Autodesk Fusion 360 part; units mm, degrees
(part 9 of 13)
  line L7144 (95.2429, -95.2347) -> (95.2261, -95.2606)
  line L7145 (95.2114, -95.2876) -> (94.7288, -95.7702)
  line L7146 (112.501, -89.0386) -> (112.377, -88.9433)
  line L7147 (112.377, -88.9433) -> (112.282, -88.819)
  line L7148 (94.6404, -95.8068) -> (94.627, -95.8068)
  line L7149 (91.2502, -96.0114) -> (91.1387, -95.9546)
  line L7150 (94.627, -95.8068) -> (94.627, -96.0518)
  line L7151 (94.7, -95.7917) -> (94.6699, -95.7981)
  line L7152 (95.248, -95.1992) -> (95.2448, -95.2212)
  line L7153 (95.2438, -95.2283) -> (95.2429, -95.2347)
  line L7154 (94.627, -96.0518) -> (92.227, -96.0518)
  line L7155 (112.957, -89.0986) -> (112.801, -89.119)
  line L7156 (91.3739, -96.031) -> (91.2502, -96.0114)
  line L7157 (95.0012, -90.6052) -> (95.0009, -90.6006)
  line L7158 (97.3892, -88.1887) -> (97.3923, -88.1852)
  line L7159 (91.4975, -96.0114) -> (91.3739, -96.031)
  line L7160 (91.6975, -95.3959) -> (91.7543, -95.5074)
  line L7161 (111.572, -88.6389) -> (111.546, -88.6222)
  line L7162 (92.227, -95.5271) -> (92.227, -95.3118)
  line L7163 (97.395, -88.1844) -> (97.4002, -88.1805)
  line L7164 (90.9797, -95.5939) -> (90.9934, -95.5074)
  line L7165 (92.227, -96.0518) -> (92.227, -95.7771)
  line L7166 (90.9934, -95.5074) -> (91.0502, -95.3959)
  line L7167 (111.546, -88.6222) -> (111.519, -88.6074)
  line L7168 (97.3923, -88.1852) -> (97.395, -88.1844)
  line L7169 (94.7079, -95.787) -> (94.7052, -95.7878)
  line L7170 (95.248, -90.679) -> (95.248, -95.1992)
  line L7171 (111.519, -88.6074) -> (111.327, -88.4154)
  line L7172 (97.5116, -88.4154) -> (95.248, -90.679)
  line L7173 (111.327, -88.4154) -> (97.5116, -88.4154)
  line L7174 (90.9745, -95.716) -> (90.9597, -95.6472)
  line L7175 (91.0502, -95.8661) -> (90.9934, -95.7546)
  line L7176 (145.432, -71.1749) -> (145.598, -71.1574)
  line L7177 (95.2451, -95.2258) -> (95.2438, -95.2283)
  line L7178 (111.578, -88.6398) -> (111.572, -88.6389)
  line L7179 (91.6975, -95.8661) -> (91.609, -95.9546)
  line L7180 (94.627, -95.5184) -> (94.998, -95.1474)
  line L7181 (91.7488, -95.7653) -> (91.6975, -95.8661)
  line L7182 (91.7555, -95.5154) -> (92.227, -95.5271)
  line L7183 (96.127, -95.3118) -> (98.527, -95.3118)
  line L7184 (111.659, -88.394) -> (112.218, -88.394)
  line L7185 (102.348, -90.1491) -> (102.359, -90.2585)
  line L7186 (98.8989, -95.787) -> (98.8962, -95.7878)
  line L7187 (99.6056, -95.0844) -> (98.9198, -95.7702)
  line L7188 (92.227, -95.3118) -> (94.627, -95.3118)
  line L7189 (112.377, -88.0947) -> (112.501, -87.9994)
  line L7190 (98.527, -95.5568) -> (98.7796, -95.5568)
  line L7191 (112.646, -87.9394) -> (112.801, -87.919)
  line L7192 (102.341, -90.3274) -> (102.326, -90.3572)
  line L7193 (95.0009, -90.6006) -> (95.0022, -90.5981)
  line L7194 (102.308, -89.4086) -> (102.419, -89.4654)
  line L7195 (91.609, -95.3074) -> (91.6975, -95.3959)
  line L7196 (102.584, -89.789) -> (102.565, -89.9126)
  line L7197 (111.401, -88.1686) -> (111.406, -88.1683)
  line L7198 (97.4303, -88.1741) -> (97.4598, -88.1654)
  line L7199 (98.527, -95.8068) -> (98.527, -96.0518)
  line L7200 (91.2502, -95.2506) -> (91.3739, -95.231)
  line L7201 (98.8314, -95.8068) -> (98.527, -95.8068)
  line L7202 (98.527, -96.0518) -> (96.127, -96.0518)
  line L7203 (100.85, -93.7382) -> (99.6422, -94.9462)
  line L7204 (98.8609, -95.7981) -> (98.8314, -95.8068)
  line L7205 (111.467, -88.202) -> (111.659, -88.394)
  line L7206 (95.0198, -90.5658) -> (95.0346, -90.5388)
  line L7207 (102.419, -90.1126) -> (102.348, -90.1491)
  line L7208 (97.4002, -88.1805) -> (97.4303, -88.1741)
  line L7209 (91.7543, -95.5074) -> (91.7555, -95.5154)
  line L7210 (111.408, -88.1696) -> (111.415, -88.1705)
  line L7211 (111.415, -88.1705) -> (111.44, -88.1872)
  line L7212 (97.4598, -88.1654) -> (111.379, -88.1654)
  line L7213 (94.998, -90.6272) -> (95.0012, -90.6052)
  line L7214 (112.222, -88.3637) -> (112.282, -88.219)
  line L7215 (112.282, -88.219) -> (112.377, -88.0947)
  line L7216 (102.508, -89.5539) -> (102.565, -89.6654)
  line L7217 (112.218, -88.394) -> (112.222, -88.3637)
  line L7218 (102.565, -89.9126) -> (102.508, -90.0241)
  line L7219 (102.359, -90.2585) -> (102.358, -90.2944)
  line L7220 (111.406, -88.1683) -> (111.408, -88.1696)
  line L7221 (100.865, -93.7112) -> (100.85, -93.7382)
  line L7222 (94.627, -95.3118) -> (94.627, -95.5184)
  line L7223 (98.527, -95.3118) -> (98.527, -95.5568)
  line L7224 (100.882, -93.6853) -> (100.865, -93.7112)
  line L7225 (95.0346, -90.5388) -> (97.3714, -88.202)
  line L7226 (90.9934, -95.7546) -> (90.9908, -95.7378)
  line L7227 (112.501, -87.9994) -> (112.646, -87.9394)
  line L7228 (100.884, -93.6718) -> (100.884, -93.6764)
  line L7229 (99.639, -95.018) -> (99.6393, -95.0226)
  line L7230 (91.4975, -95.2506) -> (91.609, -95.3074)
  line L7231 (102.508, -90.0241) -> (102.419, -90.1126)
  line L7232 (102.358, -90.2944) -> (102.357, -90.2962)
  line L7233 (102.357, -90.2962) -> (102.357, -90.2982)
  line L7234 (102.419, -89.4654) -> (102.508, -89.5539)
  line L7235 (102.357, -90.2982) -> (102.341, -90.3274)
  line L7236 (91.0502, -95.3959) -> (91.1387, -95.3074)
  line L7237 (112.801, -87.919) -> (112.957, -87.9394)
  line L7238 (99.6393, -95.0226) -> (99.638, -95.0251)
  line L7239 (102.565, -89.6654) -> (102.584, -89.789)
  line L7240 (95.0031, -90.5917) -> (95.0198, -90.5658)
  line L7241 (111.44, -88.1872) -> (111.467, -88.202)
  line L7242 (102.326, -90.3572) -> (102.324, -90.3582)
  line L7243 (111.379, -88.1654) -> (111.401, -88.1686)
  line L7244 (98.902, -95.7835) -> (98.8989, -95.787)
  line L7245 (98.891, -95.7917) -> (98.8609, -95.7981)
  line L7246 (102.324, -90.3582) -> (102.323, -90.36)
  line L7247 (99.096, -94.3086) -> (99.123, -94.3234)
  line L7248 (126.104, -71.9283) -> (126.081, -72.0939)
  line L7249 (100.884, -93.6764) -> (100.883, -93.6789)
  line L7250 (102.061, -89.4086) -> (102.184, -89.389)
  line L7251 (129.614, -81.2299) -> (129.644, -81.2338)
  line L7252 (96.127, -94.0418) -> (98.527, -94.0418)
  line L7253 (101.949, -90.1126) -> (101.861, -90.0241)
  line L7254 (102.184, -89.389) -> (102.308, -89.4086)
  line L7255 (99.6422, -94.9462) -> (99.6422, -94.996)
  line L7256 (96.127, -94.7818) -> (96.127, -94.0418)
  line L7257 (102.099, -90.1755) -> (102.061, -90.1694)
  line L7258 (129.294, -75.6781) -> (129.301, -75.7082)
  line L7259 (99.0346, -94.2868) -> (99.0566, -94.29)
  line L7260 (101.949, -89.4654) -> (102.061, -89.4086)
  line L7261 (96.127, -96.0518) -> (96.127, -95.3118)
  line L7262 (99.6422, -94.996) -> (99.639, -95.018)
  line L7263 (98.527, -94.7818) -> (96.127, -94.7818)
  line L7264 (100.637, -91.7448) -> (100.64, -91.7228)
  line L7265 (100.64, -91.7228) -> (100.64, -91.7182)
  line L7266 (125.942, -71.4415) -> (126.03, -71.5833)
  line L7267 (125.683, -71.2333) -> (125.824, -71.3229)
  line L7268 (129.286, -75.6672) -> (129.29, -75.6702)
  line L7269 (98.8962, -95.7878) -> (98.891, -95.7917)
  line L7270 (99.0637, -94.291) -> (99.0701, -94.2919)
  line L7271 (99.638, -95.0251) -> (99.6371, -95.0315)
  line L7272 (129.578, -76.0608) -> (129.591, -76.0786)
  line L7273 (100.887, -91.7966) -> (100.887, -93.6498)
  line L7274 (100.64, -91.7182) -> (100.641, -91.7157)
  line L7275 (100.659, -91.6834) -> (100.673, -91.6564)
  line L7276 (101.861, -90.0241) -> (101.804, -89.9126)
  line L7277 (98.9828, -94.5368) -> (98.527, -94.5368)
  line L7278 (129.595, -76.0844) -> (129.599, -76.0896)
  line L7279 (100.887, -93.6498) -> (100.884, -93.6718)
  line L7280 (99.0701, -94.2919) -> (99.096, -94.3086)
  line L7281 (102.323, -90.36) -> (100.887, -91.7966)
  line L7282 (101.784, -89.789) -> (101.804, -89.6654)
  line L7283 (100.637, -93.598) -> (100.637, -91.7448)
  line L7284 (129.301, -75.7082) -> (129.309, -75.7377)
  line L7285 (129.606, -76.1197) -> (129.614, -76.1492)
  line L7286 (102.104, -90.2254) -> (102.099, -90.1755)
  line L7287 (98.9198, -95.7702) -> (98.902, -95.7835)
  line L7288 (125.962, -72.3388) -> (129.273, -75.6493)
  line L7289 (101.804, -89.9126) -> (101.784, -89.789)
  line L7290 (99.3912, -94.9452) -> (98.9828, -94.5368)
  line L7291 (98.527, -94.5368) -> (98.527, -94.7818)
  line L7292 (99.6371, -95.0315) -> (99.6204, -95.0574)
  line L7293 (129.614, -76.1492) -> (129.614, -81.2299)
  line L7294 (99.0612, -94.2897) -> (99.0637, -94.291)
  line L7295 (99.0566, -94.29) -> (99.0612, -94.2897)
  line L7296 (100.642, -91.7093) -> (100.659, -91.6834)
  line L7297 (102.061, -90.1694) -> (101.949, -90.1126)
  line L7298 (129.599, -76.0896) -> (129.606, -76.1197)
  line L7299 (100.673, -91.6564) -> (102.104, -90.2254)
  line L7300 (98.527, -94.0418) -> (98.527, -94.2868)
  line L7301 (129.591, -76.0786) -> (129.594, -76.0817)
  line L7302 (99.123, -94.3234) -> (99.5172, -94.7176)
  line L7303 (129.29, -75.6729) -> (129.294, -75.6781)
  line L7304 (98.527, -94.2868) -> (99.0346, -94.2868)
  line L7305 (98.7796, -95.5568) -> (99.3912, -94.9452)
  line L7306 (99.6204, -95.0574) -> (99.6056, -95.0844)
  line L7307 (100.883, -93.6789) -> (100.882, -93.6853)
  line L7308 (99.5172, -94.7176) -> (100.637, -93.598)
  line L7309 (100.641, -91.7157) -> (100.642, -91.7093)
  line L7310 (129.594, -76.0817) -> (129.595, -76.0844)
  line L7311 (128.91, -81.9687) -> (128.889, -81.8134)
  line L7312 (129.273, -75.6493) -> (129.286, -75.6672)
  line L7313 (125.525, -71.1772) -> (125.683, -71.2333)
  line L7314 (126.984, -94.7586) -> (126.873, -94.8154)
  line L7315 (130.089, -81.8134) -> (130.069, -81.9687)
  line L7316 (126.03, -71.5833) -> (126.085, -71.7412)
  line L7317 (130.069, -81.6581) -> (130.089, -81.8134)
  line L7318 (129.913, -81.3891) -> (130.009, -81.5134)
  line L7319 (129.364, -82.3969) -> (129.334, -82.393)
  line L7320 (126.369, -94.3114) -> (126.426, -94.1999)
  line L7321 (129.309, -75.7926) -> (129.578, -76.0608)
  line L7322 (129.614, -87.0204) -> (129.611, -87.0424)
  line L7323 (127.13, -94.3114) -> (127.149, -94.435)
  line L7324 (126.349, -94.435) -> (126.369, -94.3114)
  line L7325 (129.61, -87.0495) -> (129.609, -87.0559)
  line L7326 (127.073, -94.1999) -> (127.13, -94.3114)
  line L7327 (126.629, -89.7248) -> (126.646, -89.6989)
  line L7328 (126.626, -94.8154) -> (126.514, -94.7586)
  line L7329 (130.009, -82.1134) -> (129.913, -82.2377)
  line L7330 (126.624, -94.0553) -> (126.624, -89.7603)
  line L7331 (126.627, -89.7383) -> (126.627, -89.7337)
  line L7332 (126.646, -89.6989) -> (126.661, -89.6719)
  line L7333 (129.29, -75.6702) -> (129.29, -75.6729)
  line L7334 (129.644, -82.393) -> (129.614, -82.3969)
  line L7335 (127.13, -94.5586) -> (127.073, -94.6701)
  line L7336 (126.749, -94.835) -> (126.626, -94.8154)
  line L7337 (130.009, -81.5134) -> (130.069, -81.6581)
  line L7338 (101.861, -89.5539) -> (101.949, -89.4654)
  line L7339 (126.021, -72.2502) -> (125.962, -72.3388)
  line L7340 (126.081, -72.0939) -> (126.021, -72.2502)
  line L7341 (101.804, -89.6654) -> (101.861, -89.5539)
  line L7342 (126.984, -94.1114) -> (127.073, -94.1999)
  line L7343 (129.789, -82.333) -> (129.644, -82.393)
  line L7344 (126.874, -89.8121) -> (126.874, -94.0553)
  line L7345 (129.611, -87.0424) -> (129.611, -87.047)
  line L7346 (129.309, -75.7377) -> (129.309, -75.7926)
  line L7347 (129.592, -87.0818) -> (129.578, -87.1088)
  line L7348 (125.824, -71.3229) -> (125.942, -71.4415)
  line L7349 (129.614, -82.3969) -> (129.614, -87.0204)
  line L7350 (129.611, -87.047) -> (129.61, -87.0495)
  line L7351 (129.789, -81.2938) -> (129.913, -81.3891)
  line L7352 (129.913, -82.2377) -> (129.789, -82.333)
  line L7353 (126.627, -89.7337) -> (126.629, -89.7312)
  line L7354 (126.629, -89.7312) -> (126.629, -89.7248)
  line L7355 (126.085, -71.7412) -> (126.104, -71.9074)
  line L7356 (126.369, -94.5586) -> (126.349, -94.435)
  line L7357 (126.104, -71.9074) -> (126.104, -71.9283)
  line L7358 (130.069, -81.9687) -> (130.009, -82.1134)
  line L7359 (126.874, -94.0553) -> (126.984, -94.1114)
  line L7360 (127.149, -94.435) -> (127.13, -94.5586)
  line L7361 (126.514, -94.7586) -> (126.426, -94.6701)
  line L7362 (129.609, -87.0559) -> (129.592, -87.0818)
  line L7363 (128.889, -81.8134) -> (128.91, -81.6581)
  line L7364 (127.073, -94.6701) -> (126.984, -94.7586)
  line L7365 (129.189, -82.333) -> (129.065, -82.2377)
  line L7366 (129.065, -81.3891) -> (129.189, -81.2938)
  line L7367 (126.624, -89.7603) -> (126.627, -89.7383)
  line L7368 (129.578, -87.1088) -> (126.874, -89.8121)
  line L7369 (126.873, -94.8154) -> (126.749, -94.835)
  line L7370 (129.364, -86.9686) -> (129.364, -82.3969)
  line L7371 (129.189, -81.2938) -> (129.334, -81.2338)
  line L7372 (129.065, -82.2377) -> (128.97, -82.1134)
  line L7373 (129.644, -81.2338) -> (129.789, -81.2938)
  line L7374 (126.426, -94.1999) -> (126.514, -94.1114)
  line L7375 (130.867, -72.5048) -> (130.724, -72.5904)
  line L7376 (131.186, -85.0363) -> (131.207, -85.1916)
  line L7377 (124.673, -72.222) -> (124.62, -72.0633)
  line L7378 (125.193, -71.1749) -> (125.359, -71.1574)
  line L7379 (124.892, -71.3164) -> (125.035, -71.2288)
  line L7380 (129.334, -82.393) -> (129.189, -82.333)
  line L7381 (130.729, -87.1694) -> (130.729, -87.174)
  line L7382 (130.729, -87.174) -> (130.728, -87.1765)
  line L7383 (129.364, -81.2299) -> (129.364, -76.201)
  line L7384 (130.907, -84.672) -> (131.031, -84.7673)
  line L7385 (130.907, -85.7112) -> (130.762, -85.7712)
  line L7386 (130.762, -84.612) -> (130.907, -84.672)
  line L7387 (125.173, -72.6351) -> (125.016, -72.5768)
  line L7388 (125.664, -72.5904) -> (125.505, -72.6421)
  line L7389 (129.079, -75.9119) -> (129.078, -75.9092)
  line L7390 (124.773, -71.4334) -> (124.892, -71.3164)
  line L7391 (131.207, -85.1916) -> (131.186, -85.3469)
  line L7392 (131.164, -71.9074) -> (131.163, -71.9283)
  line L7393 (128.97, -82.1134) -> (128.91, -81.9687)
  line L7394 (130.884, -71.3229) -> (131.002, -71.4415)
  line L7395 (129.075, -75.904) -> (129.068, -75.8739)
  line L7396 (125.359, -71.1574) -> (125.525, -71.1772)
  line L7397 (124.62, -72.0633) -> (124.604, -71.8969)
  line L7398 (131.126, -85.4916) -> (131.031, -85.6159)
  line L7399 (129.059, -75.7895) -> (125.787, -72.5171)
  line L7400 (125.338, -72.6572) -> (125.173, -72.6351)
  line L7401 (129.334, -81.2338) -> (129.364, -81.2299)
  line L7402 (131.145, -71.7412) -> (131.164, -71.9074)
  line L7403 (130.539, -72.6444) -> (130.539, -84.6006)
  line L7404 (130.724, -72.5904) -> (130.565, -72.6421)
  line L7405 (129.083, -75.915) -> (129.079, -75.9119)
  line L7406 (130.743, -71.2333) -> (130.884, -71.3229)
  line L7407 (128.91, -81.6581) -> (128.97, -81.5134)
  line L7408 (130.585, -71.1772) -> (130.743, -71.2333)
  line L7409 (129.096, -75.9328) -> (129.083, -75.915)
  line L7410 (129.364, -76.201) -> (129.096, -75.9328)
  line L7411 (125.505, -72.6421) -> (125.338, -72.6572)
  line L7412 (124.76, -72.365) -> (124.673, -72.222)
  line L7413 (130.762, -85.7712) -> (130.732, -85.7751)
  line L7414 (131.081, -72.2502) -> (130.988, -72.3895)
  line L7415 (130.732, -85.7751) -> (130.732, -87.1474)
  line L7416 (131.031, -85.6159) -> (130.907, -85.7112)
  line L7417 (125.035, -71.2288) -> (125.193, -71.1749)
  line L7418 (126.661, -89.6719) -> (129.364, -86.9686)
  line L7419 (126.426, -94.6701) -> (126.369, -94.5586)
  line L7420 (124.682, -71.5739) -> (124.773, -71.4334)
  line L7421 (125.787, -72.5171) -> (125.664, -72.5904)
  line L7422 (129.078, -75.9092) -> (129.075, -75.904)
  line L7423 (129.059, -75.8444) -> (129.059, -75.7895)
  line L7424 (124.876, -72.4853) -> (124.76, -72.365)
  line L7425 (124.604, -71.8969) -> (124.625, -71.731)
  line L7426 (131.186, -85.3469) -> (131.126, -85.4916)
  line L7427 (129.068, -75.8739) -> (129.059, -75.8444)
  line L7428 (124.625, -71.731) -> (124.682, -71.5739)
  line L7429 (131.14, -72.0939) -> (131.081, -72.2502)
  line L7430 (126.514, -94.1114) -> (126.624, -94.0553)
  line L7431 (131.002, -71.4415) -> (131.09, -71.5833)
  line L7432 (128.97, -81.5134) -> (129.065, -81.3891)
  line L7433 (125.016, -72.5768) -> (124.876, -72.4853)
  line L7434 (130.565, -72.6421) -> (130.539, -72.6444)
  line L7435 (130.607, -84.5916) -> (130.762, -84.612)
  line L7436 (130.988, -72.3895) -> (130.867, -72.5048)
  line L7437 (131.126, -84.8916) -> (131.186, -85.0363)
  line L7438 (130.732, -87.1474) -> (130.729, -87.1694)
  line L7439 (130.728, -87.1765) -> (130.727, -87.1829)
  line L7440 (128.2, -93.7083) -> (128.22, -93.8319)
  line L7441 (128.144, -93.5968) -> (128.2, -93.7083)
  line L7442 (127.42, -93.8319) -> (127.44, -93.7083)
  line L7443 (128.055, -93.5083) -> (128.144, -93.5968)
  line L7444 (129.664, -71.8969) -> (129.685, -71.731)
  line L7445 (127.496, -94.0671) -> (127.44, -93.9555)
  line L7446 (130.027, -85.3469) -> (130.007, -85.1916)
  line L7447 (127.945, -89.9859) -> (127.945, -93.4522)
  line L7448 (130.087, -85.4916) -> (130.027, -85.3469)
  line L7449 (127.585, -94.1555) -> (127.496, -94.0671)
  line L7450 (130.183, -85.6159) -> (130.087, -85.4916)
  line L7451 (92.227, -93.0168) -> (92.227, -92.7718)
  line L7452 (127.585, -93.5083) -> (127.695, -93.4522)
  line L7453 (128.2, -93.9555) -> (128.144, -94.0671)
  line L7454 (128.055, -94.1555) -> (127.944, -94.2124)
  line L7455 (130.539, -84.6006) -> (130.607, -84.5916)
  line L7456 (127.944, -94.2124) -> (127.82, -94.2319)
  line L7457 (127.698, -89.9121) -> (127.698, -89.9075)
  line L7458 (130.289, -84.6858) -> (130.289, -72.6427)
  line L7459 (128.22, -93.8319) -> (128.2, -93.9555)
  line L7460 (131.09, -71.5833) -> (131.145, -71.7412)
  line L7461 (130.482, -87.0956) -> (130.482, -85.7751)
  line L7462 (130.727, -87.1829) -> (130.71, -87.2088)
  line L7463 (131.163, -71.9283) -> (131.14, -72.0939)
  line L7464 (127.698, -89.9075) -> (127.699, -89.905)
  line L7465 (127.717, -89.8728) -> (127.732, -89.8457)
  line L7466 (131.031, -84.7673) -> (131.126, -84.8916)
  line L7467 (127.945, -93.4522) -> (128.055, -93.5083)
  line L7468 (130.695, -87.2358) -> (127.945, -89.9859)
  line L7469 (127.44, -93.7083) -> (127.496, -93.5968)
  line L7470 (127.695, -93.4522) -> (127.695, -89.9341)
  line L7471 (128.144, -94.0671) -> (128.055, -94.1555)
  line L7472 (127.496, -93.5968) -> (127.585, -93.5083)
  line L7473 (130.71, -87.2088) -> (130.695, -87.2358)
  line L7474 (127.695, -89.9341) -> (127.698, -89.9121)
  line L7475 (127.696, -94.2124) -> (127.585, -94.1555)
  line L7476 (130.482, -85.7751) -> (130.452, -85.7712)
  line L7477 (127.7, -89.8986) -> (127.717, -89.8728)
  line L7478 (127.699, -89.905) -> (127.7, -89.8986)
  line L7479 (130.452, -85.7712) -> (130.307, -85.7112)
  line L7480 (127.44, -93.9555) -> (127.42, -93.8319)
  line L7481 (130.087, -84.8916) -> (130.183, -84.7673)
  line L7482 (98.527, -93.5118) -> (96.127, -93.5118)
  line L7483 (96.127, -93.5118) -> (96.127, -92.7718)
  line L7484 (130.307, -85.7112) -> (130.183, -85.6159)
  line L7485 (90.2188, -92.3788) -> (90.8568, -93.0168)
  line L7486 (129.685, -71.731) -> (129.742, -71.5739)
  line L7487 (127.82, -94.2319) -> (127.696, -94.2124)
  line L7488 (127.732, -89.8457) -> (130.482, -87.0956)
  line L7489 (90.8568, -93.0168) -> (92.227, -93.0168)
  line L7490 (89.9878, -92.4954) -> (89.9839, -92.4902)
  line L7491 (130.007, -85.1916) -> (130.027, -85.0363)
  line L7492 (96.127, -92.7718) -> (98.527, -92.7718)
  line L7493 (89.9886, -92.4981) -> (89.9878, -92.4954)
  line L7494 (129.936, -72.4853) -> (129.82, -72.365)
  line L7495 (90.7436, -93.245) -> (90.7166, -93.2302)
  line L7496 (89.9688, -91.1098) -> (89.972, -91.0878)
  line L7497 (93.1076, -87.9265) -> (93.1377, -87.9201)
  line L7498 (90.7695, -93.2617) -> (90.7436, -93.245)
  line L7499 (92.227, -93.2668) -> (90.805, -93.2668)
  line L7500 (90.783, -93.2636) -> (90.7784, -93.2639)
  line L7501 (90.7166, -93.2302) -> (90.0054, -92.519)
  line L7502 (129.742, -71.5739) -> (129.833, -71.4334)
  line L7503 (130.094, -71.2288) -> (130.253, -71.1749)
  line L7504 (98.527, -92.7718) -> (98.527, -93.5118)
  line L7505 (130.253, -71.1749) -> (130.419, -71.1574)
  line L7506 (93.1024, -87.9304) -> (93.1076, -87.9265)
  line L7507 (90.7784, -93.2639) -> (90.7759, -93.2626)
  line L7508 (89.9717, -91.0832) -> (89.973, -91.0807)
  line L7509 (94.627, -92.7718) -> (94.627, -93.5118)
  line L7510 (129.68, -72.0633) -> (129.664, -71.8969)
  line L7511 (129.82, -72.365) -> (129.733, -72.222)
  line L7512 (90.0054, -91.0214) -> (93.0788, -87.948)
  line L7513 (129.833, -71.4334) -> (129.952, -71.3164)
  line L7514 (130.076, -72.5768) -> (129.936, -72.4853)
  line L7515 (129.952, -71.3164) -> (130.094, -71.2288)
  line L7516 (130.289, -72.6427) -> (130.232, -72.6351)
  line L7517 (93.1377, -87.9201) -> (93.1672, -87.9114)
  line L7518 (95.249, -87.9114) -> (96.5308, -86.6297)
  line L7519 (93.1672, -87.9114) -> (95.249, -87.9114)
  line L7520 (94.627, -93.5118) -> (92.227, -93.5118)
  line L7521 (93.0997, -87.9312) -> (93.1024, -87.9304)
  line L7522 (90.805, -93.2668) -> (90.783, -93.2636)
  line L7523 (130.027, -85.0363) -> (130.087, -84.8916)
  line L7524 (130.419, -71.1574) -> (130.585, -71.1772)
  line L7525 (89.9688, -92.4306) -> (89.9688, -91.1098)
  line L7526 (92.227, -93.5118) -> (92.227, -93.2668)
  line L7527 (89.9739, -91.0743) -> (89.9906, -91.0484)
  line L7528 (92.227, -92.7718) -> (94.627, -92.7718)
  line L7529 (93.0788, -87.948) -> (93.0966, -87.9347)
  line L7530 (89.9775, -92.4601) -> (89.9688, -92.4306)
  line L7531 (130.232, -72.6351) -> (130.076, -72.5768)
  line L7532 (89.972, -91.0878) -> (89.9717, -91.0832)
  line L7533 (129.733, -72.222) -> (129.68, -72.0633)
  line L7534 (89.9921, -92.5012) -> (89.9886, -92.4981)
  line L7535 (89.973, -91.0807) -> (89.9739, -91.0743)
  line L7536 (90.7759, -93.2626) -> (90.7695, -93.2617)
  line L7537 (93.0966, -87.9347) -> (93.0997, -87.9312)
  line L7538 (130.183, -84.7673) -> (130.289, -84.6858)
  line L7539 (89.9906, -91.0484) -> (90.0054, -91.0214)
  line L7540 (123.432, -92.4354) -> (123.528, -92.3111)
  line L7541 (120.78, -92.105) -> (120.925, -92.165)
  line L7542 (124.552, -92.7354) -> (124.532, -92.8907)
  line L7543 (96.5308, -86.6297) -> (96.4952, -86.5598)
  line L7544 (96.6405, -86.1126) -> (96.752, -86.0558)
  line L7545 (97.1107, -86.7598) -> (96.9992, -86.8166)
  line L7546 (96.4952, -86.3126) -> (96.552, -86.2011)
  line L7547 (96.8756, -86.8362) -> (96.752, -86.8166)
  line L7548 (95.3656, -88.1424) -> (95.3604, -88.1463)
  line L7549 (95.3604, -88.1463) -> (95.3303, -88.1527)
  line L7550 (120.78, -93.2642) -> (120.625, -93.2846)
  line L7551 (97.2756, -86.4362) -> (97.256, -86.5598)
  line L7552 (124.252, -93.255) -> (124.107, -93.315)
  line L7553 (96.752, -86.0558) -> (96.8756, -86.0362)
  line L7554 (96.7158, -86.7982) -> (95.3892, -88.1248)
  line L7555 (97.1107, -86.1126) -> (97.1992, -86.2011)
  line L7556 (95.3683, -88.1416) -> (95.3656, -88.1424)
  line L7557 (124.472, -93.0354) -> (124.376, -93.1597)
  line L7558 (96.552, -86.2011) -> (96.6405, -86.1126)
  line L7559 (124.107, -93.315) -> (123.952, -93.3354)
  line L7560 (97.256, -86.5598) -> (97.1992, -86.6713)
  line L7561 (123.372, -92.8907) -> (123.352, -92.7354)
  line L7562 (124.376, -92.3111) -> (124.472, -92.4354)
  line L7563 (123.952, -92.1354) -> (124.107, -92.1558)
  line L7564 (96.752, -86.8166) -> (96.7158, -86.7982)
  line L7565 (123.952, -93.3354) -> (123.797, -93.315)
  line L7566 (97.256, -86.3126) -> (97.2756, -86.4362)
  line L7567 (90.2188, -91.1616) -> (90.2188, -92.3788)
  line L7568 (123.797, -92.1558) -> (123.952, -92.1354)
  line L7569 (123.652, -92.2158) -> (123.797, -92.1558)
  line L7570 (120.925, -92.165) -> (121.049, -92.2603)
  line L7571 (121.049, -92.2603) -> (121.144, -92.3846)
  line L7572 (90.0054, -92.519) -> (89.9921, -92.5012)
  line L7573 (95.3714, -88.1381) -> (95.3683, -88.1416)
  line L7574 (96.4756, -86.4362) -> (96.4952, -86.3126)
  line L7575 (95.3008, -88.1614) -> (93.219, -88.1614)
  line L7576 (124.252, -92.2158) -> (124.376, -92.3111)
  line L7577 (121.225, -92.6846) -> (121.204, -92.8399)
  line L7578 (95.3892, -88.1248) -> (95.3714, -88.1381)
  line L7579 (96.8756, -86.0362) -> (96.9992, -86.0558)
  line L7580 (89.9839, -92.4902) -> (89.9775, -92.4601)
  line L7581 (97.1992, -86.6713) -> (97.1107, -86.7598)
  line L7582 (95.3303, -88.1527) -> (95.3008, -88.1614)
  line L7583 (97.1992, -86.2011) -> (97.256, -86.3126)
  line L7584 (124.532, -92.8907) -> (124.472, -93.0354)
  line L7585 (96.4952, -86.5598) -> (96.4756, -86.4362)
  line L7586 (96.9992, -86.0558) -> (97.1107, -86.1126)
  line L7587 (93.219, -88.1614) -> (90.2188, -91.1616)
  line L7588 (120.925, -93.2042) -> (120.78, -93.2642)
  line L7589 (96.9992, -86.8166) -> (96.8756, -86.8362)
  line L7590 (121.144, -92.9846) -> (121.049, -93.1089)
  line L7591 (121.144, -92.3846) -> (121.204, -92.5293)
  line L7592 (121.204, -92.5293) -> (121.225, -92.6846)
  line L7593 (124.376, -93.1597) -> (124.252, -93.255)
  line L7594 (124.107, -92.1558) -> (124.252, -92.2158)
  line L7595 (121.049, -93.1089) -> (120.925, -93.2042)
  line L7596 (136.044, -87.344) -> (136.056, -87.3434)
  line L7597 (137.219, -85.9102) -> (137.286, -85.9336)
  line L7598 (124.472, -92.4354) -> (124.532, -92.5801)
  line L7599 (136.257, -87.3131) -> (136.439, -87.2514)
  line L7600 (121.204, -92.8399) -> (121.144, -92.9846)
  line L7601 (120.2, -92.2603) -> (120.325, -92.165)
  line L7602 (120.045, -92.8399) -> (120.025, -92.6846)
  line L7603 (120.045, -92.5293) -> (120.105, -92.3846)
  line L7604 (136.571, -86.3883) -> (136.552, -86.4343)
  line L7605 (137.15, -85.9267) -> (137.219, -85.9102)
  line L7606 (136.571, -86.0777) -> (136.592, -86.233)
  line L7607 (135.642, -87.289) -> (135.653, -87.2926)
  line L7608 (123.372, -92.5801) -> (123.432, -92.4354)
  line L7609 (137.102, -86.2949) -> (137.103, -86.2875)
  line L7610 (135.331, -87.3466) -> (135.351, -87.2784)
  line L7611 (136.246, -87.3158) -> (136.257, -87.3131)
  line L7612 (120.105, -92.9846) -> (120.045, -92.8399)
  line L7613 (136.941, -86.8059) -> (137.005, -86.6906)
  line L7614 (137.005, -86.6906) -> (137.01, -86.6801)
  line L7615 (120.469, -92.105) -> (120.625, -92.0846)
  line L7616 (123.797, -93.315) -> (123.652, -93.255)
  line L7617 (123.352, -92.7354) -> (123.372, -92.5801)
  line L7618 (120.625, -92.0846) -> (120.78, -92.105)
  line L7619 (120.105, -92.3846) -> (120.2, -92.2603)
  line L7620 (136.416, -85.8087) -> (136.511, -85.933)
  line L7621 (136.592, -86.233) -> (136.571, -86.3883)
  line L7622 (120.325, -92.165) -> (120.469, -92.105)
  line L7623 (136.292, -85.7134) -> (136.416, -85.8087)
  line L7624 (135.475, -87.2218) -> (135.507, -87.2308)
  line L7625 (137.103, -86.2875) -> (137.104, -86.2367)
  line L7626 (123.432, -93.0354) -> (123.372, -92.8907)
  line L7627 (137.104, -86.2293) -> (137.087, -86.0475)
  line L7628 (135.331, -92.6423) -> (135.331, -87.3466)
  line L7629 (137.447, -92.1893) -> (137.427, -92.2574)
  line L7630 (137.286, -85.9336) -> (137.302, -85.9469)
  line L7631 (136.147, -85.6534) -> (136.292, -85.7134)
  line L7632 (124.532, -92.5801) -> (124.552, -92.7354)
  line L7633 (123.652, -93.255) -> (123.528, -93.1597)
  line L7634 (120.2, -93.1089) -> (120.105, -92.9846)
  line L7635 (120.325, -93.2042) -> (120.2, -93.1089)
  line L7636 (135.343, -92.6946) -> (135.331, -92.6423)
  line L7637 (137.302, -85.9469) -> (137.41, -86.055)
  line L7638 (136.957, -92.7314) -> (136.895, -92.7654)
  line L7639 (137.104, -86.2367) -> (137.104, -86.2293)
  line L7640 (137.41, -92.2784) -> (136.957, -92.7314)
  line L7641 (123.528, -93.1597) -> (123.432, -93.0354)
  line L7642 (136.511, -85.933) -> (136.571, -86.0777)
  line L7643 (136.934, -86.8108) -> (136.941, -86.8059)
  line L7644 (137.072, -86.4982) -> (137.074, -86.487)
  line L7645 (137.074, -86.487) -> (137.102, -86.2949)
  line L7646 (120.625, -93.2846) -> (120.469, -93.2642)
  line L7647 (136.922, -86.804) -> (136.934, -86.8108)
  line L7648 (136.056, -87.3434) -> (136.246, -87.3158)
  line L7649 (123.528, -92.3111) -> (123.652, -92.2158)
  line L7650 (137.01, -86.6801) -> (137.072, -86.4982)
  line L7651 (136.552, -86.4343) -> (136.922, -86.804)
  line L7652 (137.427, -92.2574) -> (137.41, -92.2784)
  line L7653 (120.025, -92.6846) -> (120.045, -92.5293)
  line L7654 (135.351, -87.2784) -> (135.405, -87.2319)
  line L7655 (135.852, -87.3365) -> (136.044, -87.344)
  line L7656 (135.507, -87.2308) -> (135.642, -87.289)
  line L7657 (135.405, -87.2319) -> (135.475, -87.2218)
  line L7658 (120.469, -93.2642) -> (120.325, -93.2042)
  line L7659 (137.447, -86.1441) -> (137.447, -92.1893)
  line L7660 (112.468, -84.0786) -> (112.624, -84.0582)
  line L7661 (112.624, -84.0582) -> (112.779, -84.0786)
  line L7662 (112.104, -84.9582) -> (112.044, -84.8135)
  line L7663 (91.502, -91.9968) -> (91.4588, -92.0815)
  line L7664 (111.685, -83.5709) -> (111.688, -83.5722)
  line L7665 (135.412, -86.3883) -> (135.392, -86.233)
  line L7666 (135.392, -86.233) -> (135.412, -86.0777)
  line L7667 (135.567, -86.6573) -> (135.472, -86.533)
  line L7668 (135.692, -85.7134) -> (135.836, -85.6534)
  line L7669 (136.147, -86.8126) -> (135.992, -86.833)
  line L7670 (111.68, -83.5712) -> (111.685, -83.5709)
  line L7671 (91.4588, -92.0815) -> (91.3703, -92.17)
  line L7672 (112.924, -85.1778) -> (112.779, -85.2378)
  line L7673 (135.457, -92.7683) -> (135.389, -92.7483)
  line L7674 (111.747, -83.6046) -> (112.299, -84.1572)
  line L7675 (112.324, -85.1778) -> (112.199, -85.0825)
  line L7676 (112.104, -84.3582) -> (112.123, -84.334)
  line L7677 (136.193, -86.7935) -> (136.147, -86.8126)
  line L7678 (94.627, -92.2418) -> (92.227, -92.2418)
  line L7679 (91.2588, -92.2268) -> (91.1352, -92.2464)
  line L7680 (135.567, -85.8087) -> (135.692, -85.7134)
  line L7681 (135.389, -92.7483) -> (135.343, -92.6946)
  line L7682 (112.324, -84.1386) -> (112.468, -84.0786)
  line L7683 (136.449, -87.2467) -> (136.56, -87.1849)
  line L7684 (111.72, -83.5898) -> (111.747, -83.6046)
  line L7685 (135.841, -87.335) -> (135.852, -87.3365)
  line L7686 (137.101, -85.9779) -> (137.15, -85.9267)
  line L7687 (137.41, -86.055) -> (137.444, -86.1173)
  line L7688 (137.444, -86.1173) -> (137.447, -86.1441)
  line L7689 (137.087, -86.0475) -> (137.101, -85.9779)
  line L7690 (135.653, -87.2926) -> (135.841, -87.335)
  line L7691 (135.836, -86.8126) -> (135.692, -86.7526)
  line L7692 (136.56, -87.1849) -> (136.569, -87.1748)
  line L7693 (112.924, -84.1386) -> (113.048, -84.2339)
  line L7694 (136.569, -87.1748) -> (136.567, -87.1671)
  line L7695 (136.868, -92.7683) -> (135.457, -92.7683)
  line L7696 (135.412, -86.0777) -> (135.472, -85.933)
  line L7697 (112.779, -84.0786) -> (112.924, -84.1386)
  line L7698 (111.688, -83.5722) -> (111.694, -83.5731)
  line L7699 (135.472, -85.933) -> (135.567, -85.8087)
  line L7700 (135.836, -85.6534) -> (135.992, -85.633)
  line L7701 (111.694, -83.5731) -> (111.72, -83.5898)
  line L7702 (135.992, -85.633) -> (136.147, -85.6534)
  line L7703 (136.567, -87.1671) -> (136.193, -86.7935)
  line L7704 (135.692, -86.7526) -> (135.567, -86.6573)
  line L7705 (92.227, -91.9968) -> (91.502, -91.9968)
  line L7706 (135.472, -86.533) -> (135.412, -86.3883)
  line L7707 (136.439, -87.2514) -> (136.449, -87.2467)
  line L7708 (136.895, -92.7654) -> (136.868, -92.7683)
  line L7709 (135.992, -86.833) -> (135.836, -86.8126)
  line L7710 (91.3703, -92.17) -> (91.2588, -92.2268)
  line L7711 (112.299, -84.1572) -> (112.324, -84.1386)
  line L7712 (97.9182, -122.179) -> (97.8258, -122.026)
  line L7713 (105.074, -138.481) -> (105.006, -138.58)
  line L7714 (103.998, -138.006) -> (103.993, -138.004)
  line L7715 (107.336, -138.577) -> (107.295, -138.513)
  line L7716 (97.8354, -121.335) -> (97.932, -121.185)
  line L7717 (147.672, -102.363) -> (147.784, -102.419)
  line L7718 (99.179, -121.194) -> (99.2735, -121.345)
  line L7719 (99.3269, -121.89) -> (99.2635, -122.056)
  line L7720 (98.9027, -120.972) -> (99.0533, -121.067)
  line L7721 (98.2114, -120.967) -> (98.3802, -120.909)
  line L7722 (99.352, -121.691) -> (99.3517, -121.713)
  line L7723 (101.752, -123.609) -> (101.758, -123.614)
  line L7724 (108.078, -129.982) -> (108.078, -138.036)
  line L7725 (97.7695, -121.857) -> (97.7521, -121.679)
  line L7726 (99.0357, -122.328) -> (98.8825, -122.419)
  line L7727 (97.8258, -122.026) -> (97.7695, -121.857)
  line L7728 (99.3321, -121.513) -> (99.352, -121.691)
  line L7729 (98.3802, -120.909) -> (98.5576, -120.891)
  line L7730 (108.042, -129.892) -> (108.076, -129.955)
  line L7731 (99.1648, -122.205) -> (99.0357, -122.328)
  line L7732 (107.955, -138.178) -> (107.877, -138.236)
  line L7733 (99.2735, -121.345) -> (99.3321, -121.513)
  line L7734 (99.3517, -121.713) -> (99.3269, -121.89)
  line L7735 (98.1913, -122.405) -> (98.0421, -122.307)
  line L7736 (104.621, -138.364) -> (104.596, -138.337)
  line L7737 (104.41, -138.191) -> (104.216, -138.084)
  line L7738 (98.8825, -122.419) -> (98.7129, -122.474)
  line L7739 (104.418, -138.197) -> (104.414, -138.193)
  line L7740 (103.988, -138.003) -> (103.832, -137.975)
  line L7741 (97.932, -121.185) -> (98.0595, -121.06)
  line L7742 (104.414, -138.193) -> (104.41, -138.191)
  line L7743 (147.929, -102.619) -> (147.949, -102.743)
  line L7744 (105.415, -138.178) -> (105.313, -138.254)
  line L7745 (104.418, -138.197) -> (104.418, -138.197)
  line L7746 (98.5352, -122.49) -> (98.3585, -122.467)
  line L7747 (103.998, -138.006) -> (103.998, -138.006)
  line L7748 (97.7521, -121.679) -> (97.7744, -121.502)
  line L7749 (97.7744, -121.502) -> (97.8354, -121.335)
  line L7750 (98.0595, -121.06) -> (98.2114, -120.967)
  line L7751 (99.0533, -121.067) -> (99.179, -121.194)
  line L7752 (98.3585, -122.467) -> (98.1913, -122.405)
  line L7753 (98.7129, -122.474) -> (98.5352, -122.49)
  line L7754 (147.872, -102.508) -> (147.929, -102.619)
  line L7755 (99.2635, -122.056) -> (99.1648, -122.205)
  line L7756 (98.5576, -120.891) -> (98.7347, -120.912)
  line L7757 (98.0421, -122.307) -> (97.9182, -122.179)
  line L7758 (147.784, -102.419) -> (147.872, -102.508)
  line L7759 (104.755, -138.513) -> (104.752, -138.508)
  line L7760 (102.752, -139.183) -> (102.81, -139.005)
  line L7761 (102.752, -139.558) -> (102.732, -139.371)
  line L7762 (104.592, -138.334) -> (104.592, -138.334)
  line L7763 (104.796, -138.577) -> (104.755, -138.513)
  line L7764 (102.81, -139.737) -> (102.752, -139.558)
  line L7765 (104.082, -140.15) -> (103.91, -140.227)
  line L7766 (103.993, -138.004) -> (103.988, -138.003)
  line L7767 (104.36, -138.842) -> (104.454, -139.005)
  line L7768 (104.817, -138.602) -> (104.796, -138.577)
  line L7769 (103.03, -140.039) -> (102.904, -139.9)
  line L7770 (102.81, -139.005) -> (102.904, -138.842)
  line L7771 (104.951, -138.625) -> (104.881, -138.633)
  line L7772 (103.832, -138.498) -> (103.91, -138.515)
  line L7773 (104.206, -138.08) -> (104.206, -138.08)
  line L7774 (102.732, -139.371) -> (102.752, -139.183)
  line L7775 (105.313, -138.254) -> (105.234, -138.314)
  line L7776 (104.234, -140.039) -> (104.082, -140.15)
  line L7777 (102.904, -138.842) -> (103.03, -138.702)
  line L7778 (104.592, -138.334) -> (104.418, -138.197)
  line L7779 (103.988, -138.003) -> (103.988, -138.003)
  line L7780 (103.91, -140.227) -> (103.726, -140.266)
  line L7781 (105.006, -138.58) -> (104.951, -138.625)
  line L7782 (103.538, -140.266) -> (103.354, -140.227)
  line L7783 (103.182, -140.15) -> (103.03, -140.039)
  line L7784 (104.512, -139.183) -> (104.532, -139.371)
  line L7785 (104.732, -138.487) -> (104.621, -138.364)
  line L7786 (104.211, -138.081) -> (104.206, -138.08)
  line L7787 (104.512, -139.558) -> (104.454, -139.737)
  line L7788 (104.216, -138.084) -> (104.211, -138.081)
  line L7789 (103.354, -140.227) -> (103.182, -140.15)
  line L7790 (104.41, -138.191) -> (104.41, -138.191)
  line L7791 (104.596, -138.337) -> (104.592, -138.334)
  line L7792 (102.904, -139.9) -> (102.81, -139.737)
  line L7793 (103.91, -138.515) -> (104.082, -138.591)
  line L7794 (104.881, -138.633) -> (104.817, -138.602)
  line L7795 (103.726, -140.266) -> (103.538, -140.266)
  line L7796 (103.182, -138.591) -> (103.354, -138.515)
  line L7797 (104.532, -139.371) -> (104.512, -139.558)
  line L7798 (103.03, -138.702) -> (103.182, -138.591)
  line L7799 (104.206, -138.08) -> (103.998, -138.006)
  line L7800 (105.234, -138.314) -> (105.074, -138.481)
  line L7801 (104.36, -139.9) -> (104.234, -140.039)
  line L7802 (104.752, -138.508) -> (104.732, -138.487)
  line L7803 (105.415, -138.178) -> (105.415, -138.178)
  line L7804 (104.454, -139.737) -> (104.36, -139.9)
  line L7805 (104.216, -138.084) -> (104.216, -138.084)
  line L7806 (103.354, -138.515) -> (103.432, -138.498)
  line L7807 (103.432, -138.498) -> (103.432, -137.976)
  line L7808 (102.052, -138.334) -> (102.052, -138.334)
  line L7809 (102.694, -138.314) -> (102.534, -138.481)
  line L7810 (102.879, -138.175) -> (102.875, -138.178)
  line L7811 (101.152, -137.963) -> (100.999, -137.961)
  line L7812 (101.448, -138.003) -> (101.23, -137.964)
  line L7813 (100.993, -137.961) -> (100.764, -137.996)
  line L7814 (102.052, -138.334) -> (101.878, -138.197)
  line L7815 (101.666, -138.08) -> (101.458, -138.006)
  line L7816 (104.454, -139.005) -> (104.512, -139.183)
  line L7817 (101.87, -138.191) -> (101.87, -138.191)
  line L7818 (101.671, -138.081) -> (101.666, -138.08)
  line L7819 (100.335, -138.178) -> (100.233, -138.254)
  line L7820 (102.215, -138.513) -> (102.212, -138.508)
  line L7821 (102.256, -138.577) -> (102.215, -138.513)
  line L7822 (101.666, -138.08) -> (101.666, -138.08)
  line L7823 (100.233, -138.254) -> (100.154, -138.314)
  line L7824 (103.08, -138.07) -> (103.08, -138.07)
  line L7825 (101.458, -138.006) -> (101.458, -138.006)
  line L7826 (99.8009, -138.633) -> (99.7371, -138.602)
  line L7827 (100.339, -138.175) -> (100.335, -138.178)
  line L7828 (101.453, -138.004) -> (101.448, -138.003)
  line L7829 (102.341, -138.633) -> (102.277, -138.602)
  line L7830 (104.082, -138.591) -> (104.234, -138.702)
  line L7831 (102.875, -138.178) -> (102.875, -138.178)
  line L7832 (103.08, -138.07) -> (102.931, -138.147)
  line L7833 (102.411, -138.625) -> (102.341, -138.633)
  line L7834 (102.875, -138.178) -> (102.773, -138.254)
  line L7835 (102.466, -138.58) -> (102.411, -138.625)
  line L7836 (101.878, -138.197) -> (101.874, -138.193)
  line L7837 (104.234, -138.702) -> (104.36, -138.842)
  line L7838 (101.878, -138.197) -> (101.878, -138.197)
  line L7839 (101.874, -138.193) -> (101.87, -138.191)
  line L7840 (101.87, -138.191) -> (101.676, -138.084)
  line L7841 (102.534, -138.481) -> (102.466, -138.58)
  line L7842 (102.773, -138.254) -> (102.694, -138.314)
  line L7843 (103.432, -137.976) -> (103.304, -137.996)
  line L7844 (103.304, -137.996) -> (103.084, -138.068)
  line L7845 (103.832, -137.975) -> (103.832, -138.498)
  line L7846 (102.081, -138.364) -> (102.056, -138.337)
  line L7847 (101.676, -138.084) -> (101.676, -138.084)
  line L7848 (102.212, -138.508) -> (102.192, -138.487)
  line L7849 (103.084, -138.068) -> (103.08, -138.07)
  line L7850 (100.391, -138.147) -> (100.339, -138.175)
  line L7851 (101.676, -138.084) -> (101.671, -138.081)
  line L7852 (102.931, -138.147) -> (102.879, -138.175)
  line L7853 (102.277, -138.602) -> (102.256, -138.577)
  line L7854 (102.056, -138.337) -> (102.052, -138.334)
  line L7855 (102.192, -138.487) -> (102.081, -138.364)
  line L7856 (99.7371, -138.602) -> (99.7164, -138.577)
  line L7857 (100.54, -138.07) -> (100.391, -138.147)
  line L7858 (97.7989, -138.175) -> (97.7947, -138.178)
  line L7859 (99.1265, -138.08) -> (98.9179, -138.006)
  line L7860 (99.3296, -138.191) -> (99.1359, -138.084)
  line L7861 (98.2245, -137.996) -> (98.0043, -138.068)
  line L7862 (97.9997, -138.07) -> (97.9997, -138.07)
  line L7863 (99.3341, -138.193) -> (99.3296, -138.191)
  line L7864 (98.9179, -138.006) -> (98.9179, -138.006)
  line L7865 (99.1314, -138.081) -> (99.1265, -138.08)
  line L7866 (100.764, -137.996) -> (100.544, -138.068)
  line L7867 (98.6901, -137.964) -> (98.6901, -137.964)
  line L7868 (100.544, -138.068) -> (100.54, -138.07)
  line L7869 (101.23, -137.964) -> (101.225, -137.964)
  line L7870 (99.1359, -138.084) -> (99.1314, -138.081)
  line L7871 (98.6901, -137.964) -> (98.685, -137.964)
  line L7872 (99.5118, -138.334) -> (99.5118, -138.334)
  line L7873 (99.7164, -138.577) -> (99.6746, -138.513)
  line L7874 (100.335, -138.178) -> (100.335, -138.178)
  line L7875 (99.1265, -138.08) -> (99.1265, -138.08)
  line L7876 (100.54, -138.07) -> (100.54, -138.07)
  line L7877 (99.5409, -138.364) -> (99.5159, -138.337)
  line L7878 (98.9079, -138.003) -> (98.9079, -138.003)
  line L7879 (98.9179, -138.006) -> (98.913, -138.004)
  line L7880 (99.1359, -138.084) -> (99.1359, -138.084)
  line L7881 (101.448, -138.003) -> (101.448, -138.003)
  line L7882 (99.9936, -138.481) -> (99.9263, -138.58)
  line L7883 (99.3296, -138.191) -> (99.3296, -138.191)
  line L7884 (98.4586, -137.961) -> (98.4586, -137.961)
  line L7885 (100.999, -137.961) -> (100.993, -137.961)
  line L7886 (100.999, -137.961) -> (100.999, -137.961)
  line L7887 (98.685, -137.964) -> (98.6121, -137.963)
  line L7888 (98.9079, -138.003) -> (98.6901, -137.964)
  line L7889 (99.5159, -138.337) -> (99.5118, -138.334)
  line L7890 (99.6718, -138.508) -> (99.6525, -138.487)
  line L7891 (98.0043, -138.068) -> (97.9997, -138.07)
  line L7892 (98.6121, -137.963) -> (98.4586, -137.961)
  line L7893 (101.458, -138.006) -> (101.453, -138.004)
  line L7894 (101.23, -137.964) -> (101.23, -137.964)
  line L7895 (99.9263, -138.58) -> (99.8714, -138.625)
  line L7896 (100.154, -138.314) -> (99.9936, -138.481)
  line L7897 (98.4586, -137.961) -> (98.4534, -137.961)
  line L7898 (99.6746, -138.513) -> (99.6718, -138.508)
  line L7899 (99.8714, -138.625) -> (99.8009, -138.633)
  line L7900 (99.3382, -138.197) -> (99.3382, -138.197)
  line L7901 (97.8514, -138.147) -> (97.7989, -138.175)
  line L7902 (101.225, -137.964) -> (101.152, -137.963)
  line L7903 (99.6525, -138.487) -> (99.5409, -138.364)
  line L7904 (98.9959, -122.926) -> (98.9959, -122.926)
  line L7905 (97.4494, -138.487) -> (97.391, -138.527)
  line L7906 (98.3186, -122.983) -> (98.3186, -122.983)
  line L7907 (99.6918, -122.342) -> (99.6918, -122.342)
  line L7908 (98.3186, -122.983) -> (98.3239, -122.984)
  line L7909 (97.2255, -138.407) -> (97.3211, -122.612)
  line L7910 (99.5118, -138.334) -> (99.3382, -138.197)
  line L7911 (97.7705, -122.741) -> (97.8953, -122.828)
  line L7912 (97.3211, -122.612) -> (97.3415, -122.544)
  line L7913 (97.5458, -122.535) -> (97.7077, -122.697)
  line L7914 (97.7947, -138.178) -> (97.7947, -138.178)
  line L7915 (97.391, -138.527) -> (97.32, -138.53)
  line L7916 (97.9002, -122.83) -> (98.0605, -122.905)
  line L7917 (98.1081, -122.926) -> (98.1081, -122.926)
  line L7918 (99.3918, -122.7) -> (99.3963, -122.697)
  line L7919 (101.914, -139.005) -> (101.972, -139.183)
  line L7920 (98.4534, -137.961) -> (98.2245, -137.996)
  line L7921 (97.7077, -122.697) -> (97.7122, -122.7)
  line L7922 (97.32, -138.53) -> (97.259, -138.493)
  line L7923 (97.543, -122.531) -> (97.5458, -122.535)
  line L7924 (97.259, -138.493) -> (97.2274, -138.43)
  line L7925 (97.3954, -122.498) -> (97.4658, -122.488)
  line L7926 (98.0605, -122.905) -> (98.1028, -122.925)
  line L7927 (97.4507, -138.485) -> (97.4494, -138.487)
  line L7928 (97.7122, -122.7) -> (97.7122, -122.7)
  line L7929 (99.2038, -122.83) -> (99.2087, -122.828)
  line L7930 (97.7122, -122.7) -> (97.7705, -122.741)
  line L7931 (97.5302, -122.518) -> (97.543, -122.531)
  line L7932 (99.2087, -122.828) -> (99.3335, -122.741)
  line L7933 (97.4536, -138.481) -> (97.4507, -138.485)
  line L7934 (97.2274, -138.43) -> (97.2255, -138.407)
  line L7935 (101.972, -139.183) -> (101.992, -139.371)
  line L7936 (98.1081, -122.926) -> (98.3186, -122.983)
  line L7937 (97.9002, -122.83) -> (97.9002, -122.83)
  line L7938 (98.7854, -122.983) -> (98.7854, -122.983)
  line L7939 (98.913, -138.004) -> (98.9079, -138.003)
  line L7940 (97.4658, -122.488) -> (97.5302, -122.518)
  line L7941 (97.6137, -138.314) -> (97.4536, -138.481)
  line L7942 (97.7947, -138.178) -> (97.6926, -138.254)
  line L7943 (97.9997, -138.07) -> (97.8514, -138.147)
  line L7944 (97.8953, -122.828) -> (97.9002, -122.83)
  line L7945 (97.6926, -138.254) -> (97.6137, -138.314)
  line L7946 (99.3382, -138.197) -> (99.3341, -138.193)
  line L7947 (98.1028, -122.925) -> (98.1081, -122.926)
  line L7948 (99.0012, -122.925) -> (99.0435, -122.905)
  line L7949 (97.3415, -122.544) -> (97.3954, -122.498)
  line L7950 (98.552, -123.004) -> (98.7801, -122.984)
  line L7951 (101.37, -138.515) -> (101.542, -138.591)
  line L7952 (145.072, -139.393) -> (145.047, -139.57)
  line L7953 (100.27, -139.737) -> (100.212, -139.558)
  line L7954 (101.972, -139.558) -> (101.914, -139.737)
  line L7955 (100.49, -138.702) -> (100.642, -138.591)
  line L7956 (101.37, -140.227) -> (101.186, -140.266)
  line L7957 (99.823, -122.235) -> (99.891, -122.256)
  line L7958 (99.0435, -122.905) -> (99.2038, -122.83)
  line L7959 (100.212, -139.183) -> (100.27, -139.005)
  line L7960 (99.5702, -122.518) -> (99.6864, -122.352)
  line L7961 (101.186, -140.266) -> (100.998, -140.266)
  line L7962 (99.7078, -122.308) -> (99.7547, -122.255)
  line L7963 (145.052, -139.193) -> (145.072, -139.371)
  line L7964 (99.7547, -122.255) -> (99.823, -122.235)
  line L7965 (101.186, -138.476) -> (101.37, -138.515)
  line L7966 (144.623, -138.652) -> (144.773, -138.747)
  line L7967 (144.455, -138.592) -> (144.623, -138.652)
  line L7968 (99.3918, -122.7) -> (99.3918, -122.7)
  line L7969 (100.814, -138.515) -> (100.998, -138.476)
  line L7970 (144.899, -138.874) -> (144.993, -139.025)
  line L7971 (99.6895, -122.347) -> (99.6918, -122.342)
  line L7972 (99.5582, -122.535) -> (99.5702, -122.518)
  line L7973 (101.542, -138.591) -> (101.694, -138.702)
  line L7974 (101.694, -138.702) -> (101.82, -138.842)
  line L7975 (101.992, -139.371) -> (101.972, -139.558)
  line L7976 (100.642, -140.15) -> (100.49, -140.039)
  line L7977 (100.212, -139.558) -> (100.192, -139.371)
  line L7978 (100.814, -140.227) -> (100.642, -140.15)
  line L7979 (99.2038, -122.83) -> (99.2038, -122.83)
  line L7980 (101.542, -140.15) -> (101.37, -140.227)
  line L7981 (145.047, -139.57) -> (144.984, -139.736)
  line L7982 (99.3335, -122.741) -> (99.3918, -122.7)
  line L7983 (101.694, -140.039) -> (101.542, -140.15)
  line L7984 (98.7854, -122.983) -> (98.9959, -122.926)
  line L7985 (145.072, -139.371) -> (145.072, -139.393)
  line L7986 (98.7801, -122.984) -> (98.7854, -122.983)
  line L7987 (101.82, -139.9) -> (101.694, -140.039)
  line L7988 (99.6864, -122.352) -> (99.6895, -122.347)
  line L7989 (98.3239, -122.984) -> (98.552, -123.004)
  line L7990 (98.9959, -122.926) -> (99.0012, -122.925)
  line L7991 (100.998, -140.266) -> (100.814, -140.227)
  line L7992 (100.364, -138.842) -> (100.49, -138.702)
  line L7993 (100.27, -139.005) -> (100.364, -138.842)
  line L7994 (100.364, -139.9) -> (100.27, -139.737)
  line L7995 (99.3963, -122.697) -> (99.5582, -122.535)
  line L7996 (101.82, -138.842) -> (101.914, -139.005)
  line L7997 (100.192, -139.371) -> (100.212, -139.183)
  line L7998 (99.6918, -122.342) -> (99.7078, -122.308)
  line L7999 (144.773, -138.747) -> (144.899, -138.874)
  line L8000 (144.255, -140.17) -> (144.078, -140.147)
  line L8001 (143.652, -138.865) -> (143.779, -138.74)
  line L8002 (118.855, -140.17) -> (118.678, -140.147)
  line L8003 (118.094, -139.182) -> (118.155, -139.015)
  line L8004 (118.988, -133.306) -> (118.997, -133.336)
  line L8005 (117.691, -131.755) -> (117.672, -131.878)
  line L8006 (117.526, -131.431) -> (117.615, -131.52)
  line L8007 (119.672, -139.393) -> (119.647, -139.57)
  line L8008 (118.531, -138.647) -> (118.7, -138.589)
  line L8009 (143.931, -138.647) -> (144.1, -138.589)
  line L8010 (100.49, -140.039) -> (100.364, -139.9)
  line L8011 (143.472, -139.359) -> (143.494, -139.182)
  line L8012 (143.489, -139.537) -> (143.472, -139.359)
  line L8013 (144.885, -139.885) -> (144.756, -140.008)
  line L8014 (101.914, -139.737) -> (101.82, -139.9)
  line L8015 (117.672, -131.631) -> (117.691, -131.755)
  line L8016 (118.978, -133.271) -> (118.982, -133.276)
  line L8017 (144.756, -140.008) -> (144.602, -140.099)
  line L8018 (118.155, -139.015) -> (118.252, -138.865)
  line L8019 (143.911, -140.085) -> (143.762, -139.987)
  line L8020 (118.511, -140.085) -> (118.362, -139.987)
  line L8021 (144.993, -139.025) -> (145.052, -139.193)
  line L8022 (144.078, -140.147) -> (143.911, -140.085)
  line L8023 (143.555, -139.015) -> (143.652, -138.865)
  line L8024 (100.998, -138.476) -> (101.186, -138.476)
  line L8025 (118.977, -133.268) -> (118.978, -133.271)
  line L8026 (118.982, -133.276) -> (118.988, -133.306)
  line L8027 (143.638, -139.859) -> (143.546, -139.706)
  line L8028 (143.546, -139.706) -> (143.489, -139.537)
  line L8029 (144.433, -140.154) -> (144.255, -140.17)
  line L8030 (144.984, -139.736) -> (144.885, -139.885)
  line L8031 (117.415, -131.374) -> (117.526, -131.431)
  line L8032 (118.678, -140.147) -> (118.511, -140.085)
  line L8033 (118.146, -139.706) -> (118.089, -139.537)
  line L8034 (119.593, -139.025) -> (119.652, -139.193)
  line L8035 (118.96, -133.247) -> (118.974, -133.265)
  line L8036 (143.762, -139.987) -> (143.638, -139.859)
  line L8037 (118.089, -139.537) -> (118.072, -139.359)
  line L8038 (100.642, -138.591) -> (100.814, -138.515)
  line L8039 (117.645, -131.931) -> (118.96, -133.247)
  line L8040 (143.494, -139.182) -> (143.555, -139.015)
  line L8041 (117.672, -131.878) -> (117.645, -131.931)
  line L8042 (117.615, -131.52) -> (117.672, -131.631)
  line L8043 (144.278, -138.571) -> (144.455, -138.592)